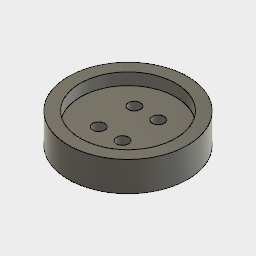
纽扣 v0 v1 (Autodesk Fusion 360 design; units mm, degrees)
Autodesk Fusion 360 part; units mm, degrees
sketch "草图1" plane through (0, 0, 0) normal (0, 1, 0) x (1, 0, 0)
  circle A0 centre (0, 0) radius 10
  circle A1 centre (0, 0) radius 8
  dimension "d3" = 2
surface "拉伸2" add extruded along (0, 1, 0) between 0 and 3 path "草图1" along A1 makes body 1
extrude "拉伸3" add sketch "草图1" along normal blind 5 separate body makes body 2
extrude "拉伸4" add sketch "草图1" along normal blind 3 contours A1 bodies 2
cylinder "圆柱体基本要素1" add diameter 2 height 20 placed x (1, 0, 0) y (0, 0, -1) z (0, 1, 0) at (25, 0, 0) separate body makes body 3
move_face "MoveFace1" to x (1, 0, 0) y (0, 1, 0) z (0, 0, 1) at (-24.9262, 0, 0) 2 faces at (25.995, 13.3333, 0.0996) (25.6415, 0, 0.2713) on bodies 3
pattern_linear "R-阵列1" count 2 spacing 4 along (1, 0, 0) count 2 spacing 6 along (0, 0, 1) of bodies 3 makes body 4 at (5.0688, 13.3333, 0.0996) makes body 5 at (1.0688, 13.3333, 6.0996) makes body 6 at (5.0688, 13.3333, 6.0996)
move_body "移动1" bodies 4 3 6 5 to x (1, 0, 0) y (0, 1, 0) z (0, 0, 1) at (-2.2168, -3.5266, -3.2244)
combine "合并1" operation cut target body 2 tool bodies 6 5 3 4
extrude "拉伸1" [rolled back] along distance -2 taper angle 0
